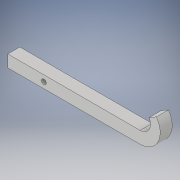
# Autodesk Inventor part: garra
Saved by Autodesk Inventor 2017 (Build 210142000, 142)
## iProperties
Created: 2019-10-07
Part Number: garra
Material: Generic
Document SubType Name: Modeling
Designer: 20171enpro0154
Density: 1 g/cm^3
Appearance: Default
Author: 20171enpro0154
Autodesk Inventor part; units mm, degrees
ref_plane "YZ Plane" through (0, 0, 0) normal (1, 0, 0) x (0, 1, 0)
ref_plane "XZ Plane" through (0, 0, 0) normal (0, 1, 0) x (-1, 0, 0)
ref_plane "XY Plane" through (0, 0, 0) normal (0, 0, 1) x (1, 0, 0)
sketch "Sketch1" plane through (0, 0, 0) normal (1, 0, 0) x (0, 1, 0)
  line L0 (0, 0) -> (15, 0)
  line L1 (15, 0) -> (15, -15)
  line L2 (15, -15) -> (0, -15)
  line L3 (0, -15) -> (0, 0)
  dimension "d1" = 15
  dimension "d2" = 15
  constraints: 8 end point, 2 parallel, 1 horizontal, 1 perpendicular
  measures "d1" distance of L1.end L2.end
  measures "d2" distance of L0.end L1.end
extrude "Extrusion1" add sketch "Sketch1" along normal blind 165
sketch "Sketch2" plane through (0, 0, 0) normal (0, 0, 1) x (1, 0, 0)
  line L0 (104.748, 28) -> (222.799, 28) construction
  line L1 (0, 15) -> (165, 15) projected
  line L2 (165, 15) -> (165, 0) projected
  line L3 (165, 15) -> (165, 53.4623) construction
  line L4 (116.7358, 25) -> (195.5126, 25) construction
  line L5 (0, 0) -> (165, 0) projected
  line L6 (176.2583, 34.5) -> (185.2344, 39.6823)
  arc A0 (165, 0) -> (185.2344, 39.6823) centre (165, 25) ccw
  arc A1 (165, 15) -> (176.2583, 34.5) centre (165, 28) ccw
  dimension "d5" = 13
  dimension "d6" = 25
  dimension "d9" = 11.2583
  dimension "d10" = 20.2344
  constraints: 9 end point, 4 point on circle, 4 point on line, 2 centre point, 2 horizontal, 1 vertical
  measures "d5" distance between parallel lines of L0 L1
  measures "d6" distance between parallel lines of L5 L4
  measures "d9" horizontal distance of A1.centre L6.start
  measures "d10" horizontal distance of L6.end A1.centre
extrude "Extrusion2" add sketch "Sketch2" against normal blind 15
sketch "Sketch3" plane through (0, 0, 0) normal (0, 0, 1) x (1, 0, 0)
  line L0 (0, 0) -> (165, 0) projected
  point P0 (45, 7.5)
hole "Hole1" at (45, 7.5, 0) direction (0, 0, -1) diameter 6 end through all
body "Solid1"
